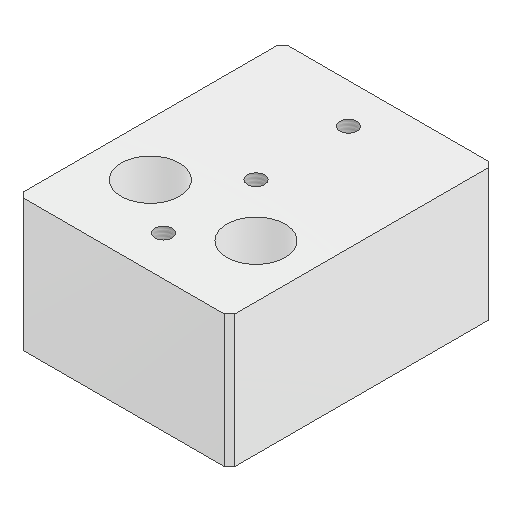
# Autodesk Inventor part: Chapa Suporte Trilho 1
Saved by Autodesk Inventor 2026.1 (Build 301233000, 233)
## iProperties
Company: Elgin
Created: 2025-09-16
Part Number: Chapa Suporte Trilho 1
Checked By: Antonio Lucas
Engr Approved By: Antonio Lucas
Material: Poliacetal WT
Document SubType Name: Modeling
Mfg Approved By: Anderson Oliveira
Designer: Willian Pinheiro
Mass: 65.3441 g
Surface Area: 100.709 cm^2
Volume: 46.6743 cm^3
Density: 1.4 g/cm^3
Appearance: Suave - Branco
Description: Chapa Suporte Trilho 1
Dimensões: 25 x 40 x 50 mm
Total: 16
Author: Willian Pinheiro
Title: Ceteva
Revision Number: 00
Autodesk Inventor part; units mm, degrees
ref_plane "YZ Plane" through (0, 0, 0) normal (1, 0, 0) x (0, 1, 0)
ref_plane "XZ Plane" through (0, 0, 0) normal (0, 1, 0) x (-1, 0, 0)
ref_plane "XY Plane" through (0, 0, 0) normal (0, 0, 1) x (1, 0, 0)
sketch "Esboço1" plane through (0, 0, 0) normal (0, 0, 1) x (1, 0, 0)
  line L0 (-28, 0) -> (28, 0) construction
  line L1 (0, -35) -> (0, 35) construction
  line L2 (-20, 25) -> (20, 25)
  line L3 (20, 25) -> (20, -25)
  line L4 (20, -25) -> (-20, -25)
  line L5 (-20, -25) -> (-20, 25)
  line L6 (-10, 25) -> (-10, -25) construction
  line L7 (10, 25) -> (10, -25) construction
  line L8 (-20, -10) -> (20, -10) construction
  point P0 (0, 0)
  point P1 (-10, -10)
  point P2 (10, -10)
  point P3 (0, -17.5)
  point P4 (0, 0)
  point P5 (0, 17.5)
  dimension "d0" = 40
  dimension "d1" = 50
  dimension "d2" = 20
  dimension "d3" = 15
  dimension "d13" = 35
  constraints: 14 end point, 9 point on line, 3 perpendicular, 3 symmetric about line, 2 parallel, 1 coincident, 1 horizontal, 2 other
  measures "d0" distance of L2.start L2.end
  measures "d1" distance of L4.end L2.start
  measures "d2" distance between parallel lines of L7 L6
  measures "d3" distance between parallel lines of L4 L8
  measures "d13" distance of point (0, 17.5) point (0, -17.5)
extrude "Extrusão1" add sketch "Esboço1" against normal blind 25
hole "Furo1" at (-10, -10, 0) at (10, -10, 0) direction (0, 0, -1) diameter 6.5 end through all counterbore diameter 11 counterbore depth 10 clearance for "Socket Head Cap Screw ISO 4762" size "M6" standard "ISO"
hole "Furo2" at (0, -17.5, 0) at (0, 0, 0) at (0, 17.5, 0) direction (0, 0, -1) diameter 3.242 depth 15 tip angle 118 thread size "M4x0.7" class "6H" standard "ISO Metric profile"
chamfer "Chanfro1" distance 1 angle 45 4 edges at (-20, -25, -12.5) (-20, 25, -12.5) (20, 25, -12.5) (20, -25, -12.5)
